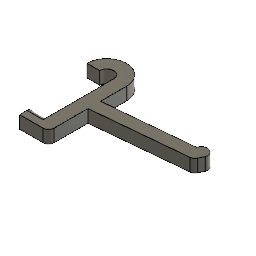
Screwdriver Hook vertical (Autodesk Fusion 360 design; units mm, degrees)
Autodesk Fusion 360 part; units mm, degrees
sketch "Sketch1" plane through (0, 0, 0) normal (0, 1, 0) x (1, 0, 0)
  circle A0 centre (0, 0) radius 7.2
  circle A1 centre (0, 0) radius 2.55
  line L0 (7.2, 0) -> (2.55, 0)
  line L1 (2.55, 0) -> (2.55, -28.2)
  line L2 (2.55, -28.2) -> (7.2, -28.2)
  line L3 (7.2, -28.2) -> (7.2, 0)
  line L4 (7.2, -28.2) -> (-3.3, -28.2)
  line L5 (-3.3, -28.2) -> (-3.3, -23.55)
  line L6 (-3.3, -23.55) -> (7.2, -23.55)
  line L7 (7.2, -23.55) -> (7.2, -28.2)
  line L8 (2.55, 0) -> (-7.2, 0)
  line L9 (7.2, -5.8) -> (7.2, -1.15)
  line L10 (7.2, -13.9742) -> (42.0463, -10.6976)
  line L11 (42.0463, -10.6976) -> (41.6194, -6.1577)
  line L12 (41.6194, -6.1577) -> (6.7731, -9.4343)
  line L13 (6.7731, -9.4343) -> (7.2, -13.9742)
  line L14 (42.0463, -10.6976) -> (37.8278, -8.7415)
  line L15 (37.8278, -8.7415) -> (40.0153, -4.024)
  line L16 (40.0153, -4.024) -> (44.2339, -5.9802)
  line L17 (44.2339, -5.9802) -> (42.0463, -10.6976)
  dimension "d1" = 14.4
  dimension "d2" = 5.1
  dimension "d3" = 4.65
  dimension "d4" = 28.2
  dimension "d5" = 10.5
  dimension "d6" = 4.65
  dimension "d16" = 35
  dimension "d17" = 4.56
  dimension "d18" = 4.65
  dimension "d19" = 5.2
  constraint coincident A0.centre A1.centre
  constraint concentric A0 A1
  constraint horizontal L0
  constraint vertical L1
  constraint horizontal L2
  constraint vertical L3
  constraint coincident A0 L0.start
  constraint coincident A1 L0.end
  constraint horizontal L4
  constraint vertical L5
  constraint horizontal L6
  constraint vertical L7
  constraint coincident A0 L8.end
  constraint perpendicular L1 L8
  constraint vertical L9
  constraint coincident L3 L9.end
  constraint perpendicular L10 L11
  constraint parallel L10 L12
  constraint parallel L11 L13
  constraint coincident L3 L10.start
  constraint perpendicular L14 L15
  constraint parallel L14 L16
  constraint parallel L15 L17
  measures "d1" diameter of A0
  measures "d2" diameter of A1
  measures "d3" horizontal distance of L1.end L2.end
  measures "d4" vertical distance of L0.start L2.end
  measures "d5" distance of L2.end L4.end
  measures "d6" distance of L2.end L6.end
  measures "d16" distance of L10.start L10.end
  measures "d17" distance of L10.start L12.end
  measures "d18" distance of L10.end L14.end
  measures "d19" distance of L10.end L16.end
extrude "Extrude1" add sketch "Sketch1" along normal blind 4.65 contours A0 A1 L0 L8 | A0 L1 L3 L6 L9 L12 L13 | A0 L0 L1 | L1 L2 L3 L4 L6 L7 | L1 L4 L5 L6 | L3 L10 L12 L14 L15 | L3 L12 L13 | L11 L12 L15 L16 L17 | L11 L12 L14 L15
fillet "Fillet1" radius 2 3 edges at (40.0153, 2.325, 4.024) (44.2339, 2.325, 5.9802) (42.0463, 2.325, 10.6976)
fillet "Fillet2" radius 2 1 edges at (7.2, 2.325, 28.2)
fillet "Fillet3" radius 2 2 edges at (-0.375, 4.65, 23.55) (-0.375, 0, 23.55)
